Autodesk Fusion 360 part; units mm, degrees
(part 2 of 2)
equation "d157 = CamInnerSeparation - CamPeg * 2"
equation "d161 = BoxOuterWidth / 2"
equation "d162 = BoxOuterHeight"
equation "d163 = BoxOuterWidth"
equation "d164 = BoxOuterHeight"
equation "d165 = BoxOuterWidth / 2"
equation "d166 = BoxOuterHeight / 2"
equation "MagnetHeight = 10 mm"
equation "MagnetWidth = 5 mm"
equation "MagnetDepth = 2 mm"
equation "d174 = MagnetWidth"
equation "d175 = MagnetHeight"
equation "d176 = MagnetWidth"
equation "d177 = MagnetHeight"
equation "d178 = BoxOuterWidth - 2 * WallThickness"
equation "d179 = BoxOuterHeight - 2 * WallThickness"
equation "d181 = WallThickness"
equation "d183 = WallThickness"
equation "d186 = WallThickness"
equation "d188 = WallThickness"
equation "d190 = 3 * WallThickness"
equation "d194 = SlitWidth"
equation "d195 = SlitHeight"
equation "d196 = WallThickness"
equation "d198 = 3 * WallThickness"
equation "d201 = WallThickness"
equation "d204 = WallThickness"
equation "CamBuffer = 10 mm"
equation "CuvetteBaseHeight = 1 mm"
equation "d218 = CuvetteBaseHeight"
named bodies: "Spectroscope Base", "Camera Mount", "Spectroscope Cap", "Camera Mount Open Center", "Spectroscope Base Modular", "Modular Variable Slit", "Modular Fixed Slit"
